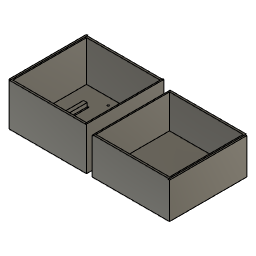
BullsEye v1 (Autodesk Fusion 360 design; units mm, degrees)
Autodesk Fusion 360 part; units mm, degrees
sketch "Sketch1" plane through (0, 0, 0) normal (0, 0, 1) x (1, 0, 0)
  line L0 (0, 0) -> (125, 0)
  line L1 (125, 0) -> (125, 125)
  line L2 (125, 125) -> (0, 125)
  line L3 (0, 125) -> (0, 0)
  dimension "d1" = 125
  dimension "d2" = 125
  constraint horizontal L0
  constraint vertical L1
  constraint horizontal L2
  constraint vertical L3
  constraint coincident L0.start L3.end
  measures "d1" distance of L0.start L0.end
  measures "d2" distance of L0.start L2.end
extrude "Extrude1" add sketch "Sketch1" along normal blind 3 makes body 1
sketch "Sketch2" plane through (0, 0, 3) normal (0, 0, 1) x (-1, 0, 0)
  line L0 (0, -125) -> (0, 0)
  line L1 (0, 0) -> (-125, 0)
  line L2 (-125, 0) -> (-125, -125)
  line L3 (-125, -125) -> (0, -125)
  line L4 (-30, -90) -> (-36, -90)
  line L5 (-36, -90) -> (-36, -30)
  line L6 (-36, -30) -> (-30, -30)
  line L7 (-30, -30) -> (-30, -90)
  line L8 (-93, -90) -> (-99, -90)
  line L9 (-99, -90) -> (-99, -30)
  line L10 (-99, -30) -> (-93, -30)
  line L11 (-93, -30) -> (-93, -90)
  dimension "d5" = 6
  dimension "d6" = 60
  dimension "d7" = 6
  dimension "d8" = 60
  dimension "d9" = 57
  dimension "d10" = 30
  dimension "d11" = 35
  dimension "d12" = 35
  constraint horizontal L4
  constraint vertical L5
  constraint horizontal L6
  constraint vertical L7
  constraint horizontal L8
  constraint vertical L9
  constraint horizontal L10
  constraint vertical L11
  measures "d5" distance of L4.start L4.end
  measures "d6" distance of L4.start L6.end
  measures "d7" distance of L8.start L8.end
  measures "d8" distance of L8.end L9.end
  measures "d9" distance of L5 L11
  measures "d10" distance of L0 L7
  measures "d11" distance of L3 L4
  measures "d12" distance of L3 L8
extrude "Extrude2" add sketch "Sketch2" along normal blind 7 contours L4 L5 L6 L7 | L8 L9 L10 L11 bodies 1
fillet "Fillet1" radius 1 1 edges at (36, 60, 3) on bodies 1
fillet "Fillet2" radius 1 1 edges at (93, 60, 3) on bodies 1
fillet "Fillet3" radius 2 6 edges at (99, 60, 3) (30, 60, 3) (33.5, 30, 3) (95.5, 30, 3) (33.5, 90, 3) (95.5, 90, 3) on bodies 1
sketch "Sketch3" plane through (0, 0, 3) normal (0, 0, 1) x (-1, 0, 0)
  line L0 (-92, -28) -> (-92, -92)
  line L1 (-92, -92) -> (-101, -92)
  line L2 (-101, -92) -> (-101, -28)
  line L3 (-101, -28) -> (-92, -28)
  line L4 (-37, -92) -> (-37, -28)
  line L5 (-37, -28) -> (-28, -28)
  line L6 (-28, -28) -> (-28, -92)
  line L7 (-28, -92) -> (-37, -92)
  line L8 (0, -125) -> (0, 0)
  line L9 (0, 0) -> (-125, 0)
  line L10 (-125, 0) -> (-125, -125)
  line L11 (-125, -125) -> (0, -125)
  circle A0 centre (-80, -110) radius 1.5
  line L12 (-80, -110) -> (-50, -110) construction
  circle A1 centre (-50, -110) radius 1.5
  dimension "d18" = 3
  dimension "d19" = 30
  dimension "d20" = 3
  dimension "d21" = 15
  dimension "d22" = 50
  constraint coincident A0.centre L12.start
  constraint parallel L11 L12
  constraint coincident L12.end A1.centre
  measures "d18" diameter of A0
  measures "d19" distance of A0.centre L12.end
  measures "d20" diameter of A1
  measures "d21" distance of L11 L12
  measures "d22" distance of L8 L12.end
extrude "Extrude3" cut sketch "Sketch3" against normal blind 7 contours A0 | A1 bodies 1
sketch "Sketch4" plane through (0, 0, 3) normal (0, 0, 1) x (-1, 0, 0)
  circle A0 centre (-50, -110) radius 1.5
  circle A1 centre (-80, -110) radius 1.5
  line L0 (-92, -28) -> (-92, -92)
  line L1 (-92, -92) -> (-101, -92)
  line L2 (-101, -92) -> (-101, -28)
  line L3 (-101, -28) -> (-92, -28)
  line L4 (-37, -92) -> (-37, -28)
  line L5 (-37, -28) -> (-28, -28)
  line L6 (-28, -28) -> (-28, -92)
  line L7 (-28, -92) -> (-37, -92)
  line L8 (0, -125) -> (0, 0)
  line L9 (0, 0) -> (-125, 0)
  line L10 (-125, 0) -> (-125, -125)
  line L11 (-125, -125) -> (0, -125)
  line L12 (-3, -3) -> (-122, -3)
  line L13 (-122, -3) -> (-122, -122)
  line L14 (-122, -122) -> (-3, -122)
  line L15 (-3, -122) -> (-3, -3)
  dimension "d25" = 3
  dimension "d26" = 3
  dimension "d27" = 3
  dimension "d28" = 3
  constraint horizontal L12
  constraint vertical L13
  constraint horizontal L14
  constraint vertical L15
  measures "d25" distance of L11 L14
  measures "d26" distance of L8 L15
  measures "d27" distance of L10 L13
  measures "d28" distance of L9 L12
extrude "Extrude4" add sketch "Sketch4" along normal blind 120 contours L8 L9 L10 L11 bodies 1
sketch "Sketch5" plane through (0, 0, 123) normal (0, 0, 1) x (-1, 0, 0)
  line L0 (-3, -3) -> (-3, -122)
  line L1 (-3, -122) -> (-122, -122)
  line L2 (-122, -122) -> (-122, -3)
  line L3 (-122, -3) -> (-3, -3)
  line L4 (-125, -125) -> (0, -125)
  line L5 (0, -125) -> (0, 0)
  line L6 (0, 0) -> (-125, 0)
  line L7 (-125, 0) -> (-125, -125)
  line L8 (0, 0) -> (-125, 0)
  line L9 (-125, 0) -> (-125, -125)
  line L10 (-125, -125) -> (0, -125)
  line L11 (0, -125) -> (0, 0)
  constraint horizontal L8
  constraint vertical L9
  constraint horizontal L10
  constraint vertical L11
  constraint coincident L4.start L7.end
  constraint coincident L5.end L6.start
extrude "Extrude5" add sketch "Sketch5" along normal blind 5 contours L0 L1 L2 L3 | L4 L5 L6 L7 L8 L9 L10 L11 bodies 1
sketch "Sketch6" plane through (0, 122, 0) normal (0, -1, 0) x (1, 0, 0)
  line L0 (3, 3) -> (122, 3)
  line L1 (122, 3) -> (122, 123)
  line L2 (122, 123) -> (3, 123)
  line L3 (-2.5, 70) -> (2.5, 70)
  line L4 (2.5, 70) -> (1, 68.5)
  line L5 (1, 68.5) -> (124, 68.5)
  line L6 (124, 68.5) -> (123, 69.5)
  line L7 (123, 69.5) -> (126.5, 69.5)
  constraint horizontal L3
  constraint perpendicular L1 L5
  constraint perpendicular L4 L6
  constraint perpendicular L1 L7
split "Split1" by curves path "Sketch6" along L3 L4 L5 L6 L7 bodies 1 makes body 2 at (58.3624, 36.1675, 0)
move_body "Move1" bodies 1 to x (-1, 0, 0) y (0, 1, 0) z (0, 0, -1) at (259.0991, 90, 129)
move_body "Move2" bodies 1 to x (1, 0, 0) y (0, 1, 0) z (0, 0, 1) at (0, 0, -1)
move_body "Move3" bodies 1 to x (1, 0, 0) y (0, 1, 0) z (0, 0, 1) at (0, -90, 0)
